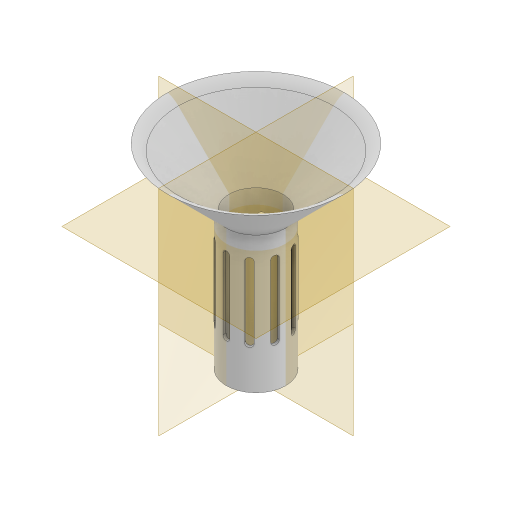
# Autodesk Inventor part: воронка
Saved by Autodesk Inventor 2023.2 (Build 272271030, 271C)
## iProperties
Created: 2025-04-19
Part Number: воронка
Material: Типовые
Document SubType Name: Modeling
Designer: Коноваленко
Density: 1 g/cm^3
Appearance: По умолчанию
Author: Коноваленко
Autodesk Inventor part; units mm, degrees
sketch "Эскиз1" plane through (0, 0, 0) normal (0, 0, 1) x (1, 0, 0)
  line L0 (0, 22.5937) -> (0, -11.0157) construction
  line L1 (88.3787, 75.9072) -> (27.5, 15.0285)
  line L2 (27.5, 15.0285) -> (27.5, -126.2141)
  line L3 (27.5, -126.2141) -> (30.5, -126.2141)
  line L4 (30.5, -126.2141) -> (30.5, 13.7859)
  line L5 (30.5, 13.7859) -> (90.5, 73.7859)
  line L6 (90.5, 73.7859) -> (88.3787, 75.9072)
  point P0 (0, 0)
  point P1 (57.9393, 45.4679)
  dimension "d0" = 3
  dimension "d1" = 3
  dimension "d3" = 27.5
  dimension "d7" = 140
  dimension "d23" = 135
  dimension "d24" = 60
  constraints: 15 end point, 3 perpendicular, 2 vertical, 1 midpoint, 1 parallel, 1 point on line
  measures "d0" distance between parallel lines of L4 L2
  measures "d1" distance from line of L5 point (57.939, 45.468)
  measures "d3" distance between parallel lines of L2 L0
  measures "d7" distance of L3.end L4.end
  measures "d23" angle of L4 L5
  measures "d24" horizontal distance of L4.end L5.end
revolve "Вращение1" add sketch "Эскиз1" angle 360 about axis through (0, 22.5937, 0) along (0, -1, 0)
fillet "Сопряжение1" radius 26.5 1 edges at (-88.3787, 75.9072, 0)
sketch "Эскиз2" plane through (0, 0, 0) normal (0, 0, 1) x (1, 0, 0)
  line L0 (3.5, -86.2141) -> (-3.5, -86.2141)
  line L1 (-3.5, -86.2141) -> (-3.5, -6.2141)
  line L2 (-3.5, -6.2141) -> (3.5, -6.2141)
  line L3 (3.5, -6.2141) -> (3.5, -86.2141)
  line L4 (3.5, -86.2141) -> (-3.5, -6.2141) construction
  line L5 (-3.5, -86.2141) -> (3.5, -6.2141) construction
  line L6 (-27.5, -126.2141) -> (27.5, -126.2141) projected
  line L7 (0, 25.2475) -> (0, -151.4853) projected
  circle A0 centre (0, -9.7141) radius 3.5
  circle A1 centre (0, -82.7141) radius 3.5
  point P0 (0, 0)
  point P1 (0, -46.2141)
  point P2 (-3.5, -9.7141)
  point P3 (-3.5, -82.7141)
  point P4 (3.5, -82.7141)
  point P5 (3.5, -9.7141)
  dimension "d8" = 7
  dimension "d9" = 80
  dimension "d10" = 40
  constraints: 12 end point, 4 tangent, 3 point on line, 2 centre point, 2 midpoint, 2 parallel, 1 horizontal, 1 perpendicular
  measures "d8" distance of L1.end L2.end
  measures "d9" distance of L2.end L0.start
  measures "d10" distance between parallel lines of L6 L0
extrude "Выдавливание1" cut sketch "Эскиз2" along normal mid plane 67 contours A1 L7 | L7 A1 | A1 L7 A0 L3 | A1 L1 A0 L7 | A0 L7 | A0 L7
pattern_circular "Круговой массив2" count 10 over 360 about axis through (0, -55.5928, 0) along (0, -1, 0) of "Выдавливание1"
